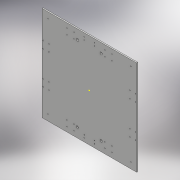
# Autodesk Inventor part: 上层板
Saved by Autodesk Inventor 2017 (Build 210142000, 142)
## iProperties
Part Number: 上层板
Material: 常规
Document SubType Name: Modeling
Designer: PANDA
Density: 1 g/cm^3
Appearance: 默认
Author: PANDA
Autodesk Inventor part; units mm, degrees
ref_plane "YZ Plane" through (0, 0, 0) normal (1, 0, 0) x (0, 1, 0)
ref_plane "XZ Plane" through (0, 0, 0) normal (0, 1, 0) x (-1, 0, 0)
ref_plane "XY Plane" through (0, 0, 0) normal (0, 0, 1) x (1, 0, 0)
sketch "草图1" plane through (0, 0, 0) normal (0, 1, 0) x (-1, 0, 0)
  line L0 (200, 200) -> (-200, 200)
  line L1 (-200, 200) -> (-200, -200)
  line L2 (-200, -200) -> (200, -200)
  line L3 (200, -200) -> (200, 200)
  point P0 (0, 0)
  dimension "d0" = 400
  dimension "d1" = 400
  constraints: 8 end point, 2 parallel, 1 horizontal, 1 perpendicular
  measures "d0" distance of L2.end L1.end
  measures "d1" distance of L1.end L0.end
extrude "拉伸1" add sketch "草图1" along normal blind 5
sketch "草图2" plane through (0, 5, 0) normal (0, 1, 0) x (1, 0, 0)
  circle A0 centre (175, 175) radius 1.8
  point P0 (0, 0)
  dimension "d4" = 3.6
  constraints: 1 centre point
  measures "d4" diameter of A0
extrude "拉伸2" cut sketch "草图2" against normal through all
sketch "草图3" plane through (0, 5, 0) normal (0, 1, 0) x (1, 0, 0)
  circle A0 centre (175, -175) radius 1.8
  point P0 (0, 0)
  dimension "d7" = 3.6
  constraints: 1 centre point
  measures "d7" diameter of A0
extrude "拉伸3" cut sketch "草图3" against normal through all
sketch "草图4" plane through (0, 0, 0) normal (0, -1, 0) x (1, 0, 0)
  circle A0 centre (-175, 175) radius 1.8
  point P0 (0, 0)
  dimension "d10" = 3.6
  constraints: 1 centre point
  measures "d10" diameter of A0
extrude "拉伸4" cut sketch "草图4" against normal through all
sketch "草图5" plane through (0, 0, 0) normal (0, -1, 0) x (1, 0, 0)
  circle A0 centre (-175, -175) radius 1.8
  point P0 (0, 0)
  dimension "d13" = 3.6
  constraints: 1 centre point
  measures "d13" diameter of A0
extrude "拉伸5" cut sketch "草图5" against normal through all
sketch "草图8" plane through (0, 5, 0) normal (0, 1, 0) x (1, 0, 0)
  circle A0 centre (-21.4, 185) radius 1.8
  point P0 (0, 0)
  dimension "d24" = 3.6
  constraints: 1 centre point
  measures "d24" diameter of A0
extrude "拉伸8" cut sketch "草图8" against normal through all
sketch "草图9" plane through (0, 5, 0) normal (0, 1, 0) x (1, 0, 0)
  circle A0 centre (21.4, 185) radius 1.8
  point P0 (0, 0)
  dimension "d27" = 3.6
  constraints: 1 centre point
  measures "d27" diameter of A0
extrude "拉伸9" cut sketch "草图9" against normal through all
sketch "草图10" plane through (0, 5, 0) normal (0, 1, 0) x (1, 0, 0)
  circle A0 centre (-21.4, 173) radius 1.8
  point P0 (0, 0)
  dimension "d30" = 3.6
  constraints: 1 centre point
  measures "d30" diameter of A0
extrude "拉伸10" cut sketch "草图10" against normal through all
sketch "草图11" plane through (0, 5, 0) normal (0, 1, 0) x (1, 0, 0)
  circle A0 centre (21.4, 173) radius 1.8
  point P0 (0, 0)
  dimension "d33" = 3.6
  constraints: 1 centre point
  measures "d33" diameter of A0
extrude "拉伸11" cut sketch "草图11" against normal through all
sketch "草图12" plane through (0, 5, 0) normal (0, 1, 0) x (1, 0, 0)
  circle A0 centre (21.4, -173) radius 1.8
  point P0 (0, 0)
  dimension "d36" = 3.6
  constraints: 1 centre point
  measures "d36" diameter of A0
extrude "拉伸12" cut sketch "草图12" against normal through all
sketch "草图13" plane through (0, 5, 0) normal (0, 1, 0) x (1, 0, 0)
  circle A0 centre (21.4, -185) radius 1.8
  point P0 (0, 0)
  dimension "d39" = 3.6
  constraints: 1 centre point
  measures "d39" diameter of A0
extrude "拉伸13" cut sketch "草图13" against normal through all
sketch "草图14" plane through (0, 5, 0) normal (0, 1, 0) x (1, 0, 0)
  circle A0 centre (-21.4, -185) radius 1.8
  point P0 (0, 0)
  dimension "d42" = 3.6
  constraints: 1 centre point
  measures "d42" diameter of A0
extrude "拉伸14" cut sketch "草图14" against normal through all
sketch "草图15" plane through (0, 5, 0) normal (0, 1, 0) x (1, 0, 0)
  circle A0 centre (-21.4, -173) radius 1.8
  point P0 (0, 0)
  dimension "d45" = 3.6
  constraints: 1 centre point
  measures "d45" diameter of A0
extrude "拉伸15" cut sketch "草图15" against normal through all
sketch "草图16" plane through (0, 5, 0) normal (0, 1, 0) x (1, 0, 0)
  circle A0 centre (50, 160) radius 5
  point P0 (0, 0)
  dimension "d48" = 10
  constraints: 1 centre point
  measures "d48" diameter of A0
extrude "拉伸16" cut sketch "草图16" against normal through all
sketch "草图17" plane through (0, 0, 0) normal (0, -1, 0) x (1, 0, 0)
  circle A0 centre (-50, 160) radius 5
  point P0 (0, 0)
  dimension "d51" = 10
  constraints: 1 centre point
  measures "d51" diameter of A0
extrude "拉伸17" cut sketch "草图17" against normal through all
sketch "草图18" plane through (0, 0, 0) normal (0, -1, 0) x (1, 0, 0)
  circle A0 centre (-50, -160) radius 5
  point P0 (0, 0)
  dimension "d54" = 10
  constraints: 1 centre point
  measures "d54" diameter of A0
extrude "拉伸18" cut sketch "草图18" against normal through all
sketch "草图19" plane through (0, 0, 0) normal (0, -1, 0) x (1, 0, 0)
  circle A0 centre (50, 160) radius 5
  point P0 (0, 0)
  dimension "d57" = 10
  constraints: 1 centre point
  measures "d57" diameter of A0
extrude "拉伸19" cut sketch "草图19" against normal through all
sketch "草图20" plane through (0, 5, 0) normal (0, 1, 0) x (1, 0, 0)
  point P0 (0, 0)
sketch "草图21" plane through (0, 5, 0) normal (0, 1, 0) x (1, 0, 0)
  point P0 (0, 0)
sketch "草图22" plane through (0, 5, 0) normal (0, 1, 0) x (1, 0, 0)
  circle A0 centre (195, -85) radius 1.8
  point P0 (0, 0)
  dimension "d60" = 3.6
  constraints: 1 centre point
  measures "d60" diameter of A0
extrude "拉伸20" cut sketch "草图22" against normal through all
sketch "草图23" plane through (0, 5, 0) normal (0, 1, 0) x (1, 0, 0)
  circle A0 centre (171, -85) radius 1.8
  point P0 (0, 0)
  dimension "d63" = 3.6
  constraints: 1 centre point
  measures "d63" diameter of A0
extrude "拉伸21" cut sketch "草图23" against normal through all
sketch "草图27" plane through (0, 5, 0) normal (0, 1, 0) x (1, 0, 0)
  circle A0 centre (-195, 85) radius 1.8
  point P0 (0, 0)
  dimension "d75" = 3.6
  constraints: 1 centre point
  measures "d75" diameter of A0
extrude "拉伸25" cut sketch "草图27" against normal through all
sketch "草图28" plane through (0, 5, 0) normal (0, 1, 0) x (1, 0, 0)
  circle A0 centre (-171, 85) radius 1.8
  point P0 (0, 0)
  dimension "d78" = 3.6
  constraints: 1 centre point
  measures "d78" diameter of A0
extrude "拉伸26" cut sketch "草图28" against normal through all
sketch "草图30" plane through (0, 0, 0) normal (0, -1, 0) x (1, 0, 0)
  circle A0 centre (171, 55) radius 1.8
  point P0 (0, 0)
  dimension "d85" = 3.6
  constraints: 1 centre point
  measures "d85" diameter of A0
extrude "拉伸27" cut sketch "草图30" against normal through all
sketch "草图31" plane through (0, 0, 0) normal (0, -1, 0) x (1, 0, 0)
  circle A0 centre (195, 55) radius 1.8
  point P0 (0, 0)
  dimension "d88" = 3.6
  constraints: 1 centre point
  measures "d88" diameter of A0
extrude "拉伸28" cut sketch "草图31" against normal through all
sketch "草图32" plane through (0, 0, 0) normal (0, -1, 0) x (1, 0, 0)
  circle A0 centre (-195, -55) radius 1.8
  point P0 (0, 0)
  dimension "d91" = 3.6
  constraints: 1 centre point
  measures "d91" diameter of A0
extrude "拉伸29" cut sketch "草图32" against normal through all
sketch "草图33" plane through (0, 0, 0) normal (0, -1, 0) x (1, 0, 0)
  circle A0 centre (-171, 55) radius 1.8
  point P0 (0, 0)
  dimension "d94" = 3.6
  constraints: 1 centre point
  measures "d94" diameter of A0
extrude "拉伸30" cut sketch "草图33" against normal through all
sketch "草图34" plane through (0, 0, 0) normal (0, -1, 0) x (1, 0, 0)
  circle A0 centre (-171, -55) radius 1.8
  point P0 (0, 0)
  dimension "d97" = 3.6
  constraints: 1 centre point
  measures "d97" diameter of A0
extrude "拉伸31" cut sketch "草图34" against normal through all
sketch "草图35" plane through (0, 0, 0) normal (0, -1, 0) x (1, 0, 0)
  circle A0 centre (-195, 55) radius 1.8
  point P0 (0, 0)
  dimension "d100" = 3.6
  constraints: 1 centre point
  measures "d100" diameter of A0
extrude "拉伸32" cut sketch "草图35" against normal through all
sketch "草图36" plane through (0, 0, 0) normal (0, -1, 0) x (1, 0, 0)
  circle A0 centre (-171, 85) radius 1.8
  point P0 (0, 0)
  dimension "d103" = 3.6
  constraints: 1 centre point
  measures "d103" diameter of A0
extrude "拉伸33" cut sketch "草图36" against normal through all
sketch "草图37" plane through (0, 0, 0) normal (0, -1, 0) x (1, 0, 0)
  circle A0 centre (-195, 85) radius 1.8
  point P0 (0, 0)
  dimension "d106" = 3.6
  constraints: 1 centre point
  measures "d106" diameter of A0
extrude "拉伸34" cut sketch "草图37" against normal through all
sketch "草图38" plane through (0, 0, 0) normal (0, -1, 0) x (1, 0, 0)
  circle A0 centre (195, -55) radius 1.8
  point P0 (0, 0)
  dimension "d109" = 3.6
  constraints: 1 centre point
  measures "d109" diameter of A0
extrude "拉伸35" cut sketch "草图38" against normal through all
sketch "草图39" plane through (0, 0, 0) normal (0, -1, 0) x (1, 0, 0)
  circle A0 centre (171, -55) radius 1.8
  point P0 (0, 0)
  dimension "d112" = 3.6
  constraints: 1 centre point
  measures "d112" diameter of A0
extrude "拉伸36" cut sketch "草图39" against normal through all
sketch "草图40" plane through (0, 0, 0) normal (0, -1, 0) x (1, 0, 0)
  circle A0 centre (171, -85) radius 1.8
  point P0 (0, 0)
  dimension "d115" = 3.6
  constraints: 1 centre point
  measures "d115" diameter of A0
extrude "拉伸37" cut sketch "草图40" against normal through all
sketch "草图41" plane through (0, 0, 0) normal (0, -1, 0) x (1, 0, 0)
  circle A0 centre (195, -85) radius 1.8
  point P0 (0, 0)
  dimension "d118" = 3.6
  constraints: 1 centre point
  measures "d118" diameter of A0
extrude "拉伸38" cut sketch "草图41" against normal through all
sketch "草图42" plane through (0, 0, 0) normal (0, -1, 0) x (1, 0, 0)
  circle A0 centre (65, 156) radius 1.8
  point P0 (0, 0)
  dimension "d121" = 3.6
  constraints: 1 centre point
  measures "d121" diameter of A0
extrude "拉伸39" cut sketch "草图42" against normal through all
sketch "草图43" plane through (0, 0, 0) normal (0, -1, 0) x (1, 0, 0)
  circle A0 centre (95, 156) radius 1.8
  point P0 (0, 0)
  dimension "d124" = 3.6
  constraints: 1 centre point
  measures "d124" diameter of A0
extrude "拉伸40" cut sketch "草图43" against normal through all
sketch "草图44" plane through (0, 0, 0) normal (0, -1, 0) x (1, 0, 0)
  circle A0 centre (65, 180) radius 1.8
  point P0 (0, 0)
  dimension "d127" = 3.6
  constraints: 1 centre point
  measures "d127" diameter of A0
extrude "拉伸41" cut sketch "草图44" against normal through all
sketch "草图45" plane through (0, 5, 0) normal (0, 1, 0) x (1, 0, 0)
  circle A0 centre (95, -180) radius 1.8
  point P0 (0, 0)
  dimension "d130" = 3.6
  constraints: 1 centre point
  measures "d130" diameter of A0
extrude "拉伸42" cut sketch "草图45" against normal through all
sketch "草图46" plane through (0, 0, 0) normal (0, -1, 0) x (1, 0, 0)
  circle A0 centre (65, -156) radius 1.8
  point P0 (0, 0)
  dimension "d133" = 3.6
  constraints: 1 centre point
  measures "d133" diameter of A0
extrude "拉伸43" cut sketch "草图46" against normal through all
sketch "草图47" plane through (0, 0, 0) normal (0, -1, 0) x (1, 0, 0)
  circle A0 centre (95, -156) radius 1.8
  point P0 (0, 0)
  dimension "d136" = 3.6
  constraints: 1 centre point
  measures "d136" diameter of A0
extrude "拉伸44" cut sketch "草图47" against normal through all
sketch "草图48" plane through (0, 0, 0) normal (0, -1, 0) x (1, 0, 0)
  circle A0 centre (65, -180) radius 1.8
  point P0 (0, 0)
  dimension "d139" = 3.6
  constraints: 1 centre point
  measures "d139" diameter of A0
extrude "拉伸45" cut sketch "草图48" against normal through all
sketch "草图49" plane through (0, 0, 0) normal (0, -1, 0) x (1, 0, 0)
  circle A0 centre (95, -180) radius 1.8
  point P0 (0, 0)
  dimension "d142" = 3.6
  constraints: 1 centre point
  measures "d142" diameter of A0
extrude "拉伸46" cut sketch "草图49" against normal through all
sketch "草图50" plane through (0, 0, 0) normal (0, -1, 0) x (1, 0, 0)
  circle A0 centre (-95, 156) radius 1.8
  point P0 (0, 0)
  dimension "d145" = 3.6
  constraints: 1 centre point
  measures "d145" diameter of A0
extrude "拉伸47" cut sketch "草图50" against normal through all
sketch "草图51" plane through (0, 0, 0) normal (0, -1, 0) x (1, 0, 0)
  circle A0 centre (-65, 156) radius 1.8
  point P0 (0, 0)
  dimension "d148" = 3.6
  constraints: 1 centre point
  measures "d148" diameter of A0
extrude "拉伸48" cut sketch "草图51" against normal through all
sketch "草图52" plane through (0, 0, 0) normal (0, -1, 0) x (1, 0, 0)
  circle A0 centre (-95, 180) radius 1.8
  point P0 (0, 0)
  dimension "d151" = 3.6
  constraints: 1 centre point
  measures "d151" diameter of A0
extrude "拉伸49" cut sketch "草图52" against normal through all
sketch "草图53" plane through (0, 0, 0) normal (0, -1, 0) x (1, 0, 0)
  circle A0 centre (-65, 180) radius 1.8
  point P0 (0, 0)
  dimension "d154" = 3.6
  constraints: 1 centre point
  measures "d154" diameter of A0
extrude "拉伸50" cut sketch "草图53" against normal through all
sketch "草图54" plane through (0, 0, 0) normal (0, -1, 0) x (1, 0, 0)
  circle A0 centre (-65, -156) radius 1.8
  point P0 (0, 0)
  dimension "d157" = 3.6
  constraints: 1 centre point
  measures "d157" diameter of A0
extrude "拉伸51" cut sketch "草图54" against normal through all
sketch "草图55" plane through (0, 0, 0) normal (0, -1, 0) x (1, 0, 0)
  circle A0 centre (-65, -180) radius 1.8
  point P0 (0, 0)
  dimension "d160" = 3.6
  constraints: 1 centre point
  measures "d160" diameter of A0
extrude "拉伸52" cut sketch "草图55" against normal through all
sketch "草图56" plane through (0, 0, 0) normal (0, -1, 0) x (1, 0, 0)
  circle A0 centre (-95, -156) radius 1.8
  point P0 (0, 0)
  dimension "d163" = 3.6
  constraints: 1 centre point
  measures "d163" diameter of A0
extrude "拉伸53" cut sketch "草图56" against normal through all
sketch "草图57" plane through (0, 0, 0) normal (0, -1, 0) x (1, 0, 0)
  circle A0 centre (-95, -180) radius 1.8
  point P0 (0, 0)
  dimension "d166" = 3.6
  constraints: 1 centre point
  measures "d166" diameter of A0
extrude "拉伸54" cut sketch "草图57" against normal through all
sketch "草图58" plane through (0, 0, 0) normal (0, -1, 0) x (1, 0, 0)
  point P0 (0, 0)
